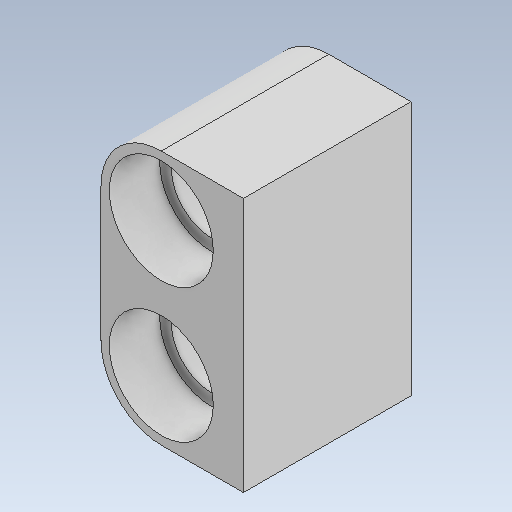
# Autodesk Inventor part: suporte sensor de cor
Saved by Autodesk Inventor 2020 (Build 240168000, 168)
## iProperties
Created: 2020-04-24
Part Number: suporte sensor de cor
Material: Genérico
Document SubType Name: Modeling
Designer: gi-se
Density: 1 g/cm^3
Appearance: Padrão
Author: gi-se
Autodesk Inventor part; units mm, degrees
ref_plane "YZ Plane" through (0, 0, 0) normal (1, 0, 0) x (0, 1, 0)
ref_plane "XZ Plane" through (0, 0, 0) normal (0, 1, 0) x (-1, 0, 0)
ref_plane "XY Plane" through (0, 0, 0) normal (0, 0, 1) x (1, 0, 0)
sketch "Esboço1" plane through (0, 0, 0) normal (0, 0, 1) x (1, 0, 0)
  circle A0 centre (0, 51.501) radius 2.4 projected
  line L0 (4.9, 66.501) -> (4.9, -3.499) projected
  line L1 (-3.6, 3.501) -> (-3.6, 59.501) projected
  arc A1 (0, 55.101) -> (-3.6, 51.501) centre (0, 51.501) ccw
  circle A2 centre (0, 43.501) radius 2.4 projected
  arc A3 (-3.6, 43.501) -> (0, 39.901) centre (0, 43.501) ccw
  line L2 (4.9, 55.101) -> (0, 55.101)
  line L3 (0, 55.101) -> (0, 39.901)
  line L4 (0, 39.901) -> (4.9, 39.901)
  line L5 (4.9, 39.901) -> (4.9, 55.101)
  point P0 (0, 0)
  constraints: 8 end point, 4 point on circle, 3 point on line, 2 centre point, 2 coincident, 2 parallel, 2 tangent, 1 horizontal, 1 perpendicular
extrude "Extrusão1" add sketch "Esboço1" along normal blind 10 contours A0 L3 L2 L0 L4 A2 | A0 L3 A2 A3 L1 A1
sketch "Esboço2" plane through (0, 0, 10) normal (0, 0, 1) x (1, 0, 0)
  circle A0 centre (0, 43.501) radius 3.1 projected
  circle A1 centre (0, 51.501) radius 3.1 projected
  point P0 (0, 0)
extrude "Extrusão2" cut sketch "Esboço2" against normal blind 3
sketch "Esboço3" plane through (0, 0, 0) normal (0, 0, -1) x (-1, 0, 0)
  circle A0 centre (0, 51.501) radius 3.1 projected
  circle A1 centre (0, 51.501) radius 2.4 projected
  circle A2 centre (0, 43.501) radius 3.1 projected
  circle A3 centre (0, 43.501) radius 2.4 projected
  point P0 (0, 0)
extrude "Extrusão3" cut sketch "Esboço3" against normal blind 1 contours A0 | A1 | A2 | A3
